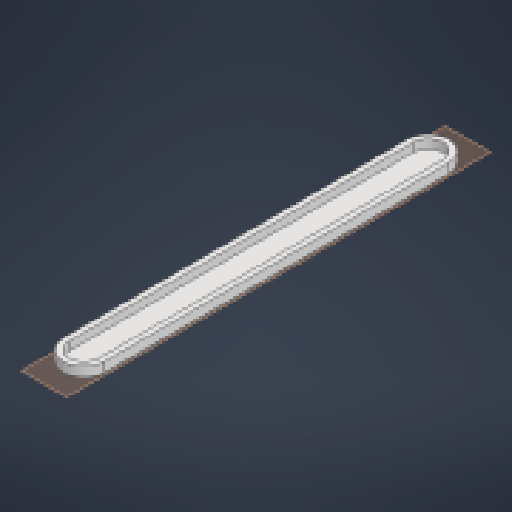
# Autodesk Inventor part: wiper_outside
Saved by Autodesk Inventor 2026.2 (Build 302298000, 298)
## iProperties
Created: 2026-04-07
Part Number: wiper_outside
Material: ABS Plastic
Document SubType Name: Modeling
Designer: Tathagata Sikdar
Density: 1.06 g/cm^3
Appearance: Smooth - White
Author: Tathagata Sikdar
Autodesk Inventor part; units mm, degrees
ref_plane "YZ Plane" through (0, 0, 0) normal (1, 0, 0) x (0, 1, 0)
ref_plane "XZ Plane" through (0, 0, 0) normal (0, 1, 0) x (-1, 0, 0)
ref_plane "XY Plane" through (0, 0, 0) normal (0, 0, 1) x (1, 0, 0)
ref_plane "Work Plane1" through (-54.4323, -35.9721, 73.855) normal (0, 1, 0) x (-1, 0, 0)
sketch "Sketch1" plane through (-54.4323, -35.9721, 73.855) normal (0, 1, 0) x (-1, 0, 0)
  arc A0 (7.2, 60.25) -> (-7.2, 60.25) centre (0, 60.25) ccw projected
  line L0 (-7.2, -60.25) -> (-7.2, 60.25) projected
  arc A1 (-7.2, -60.25) -> (7.2, -60.25) centre (0, -60.25) ccw projected
  line L1 (7.2, 60.25) -> (7.2, -60.25) projected
  arc A2 (-5.2, -60.25) -> (5.2, -60.25) centre (0, -60.25) ccw projected
  line L2 (-5.2, -60.25) -> (-5.2, 60.25) projected
  line L3 (5.2, 60.25) -> (5.2, -60.25) projected
  arc A3 (5.2, 60.25) -> (-5.2, 60.25) centre (0, 60.25) ccw projected
  point P0 (-54.4323, -73.855)
extrude "Extrusion1" add sketch "Sketch1" along normal blind 0.4 contours L1 A1 L0 A0 | L2 A3 L3 A2
sketch "Sketch2" plane through (-54.4323, -35.5721, 73.855) normal (0, 1, 0) x (1, 0, 0)
  arc A0 (-7.2, -60.25) -> (7.2, -60.25) centre (0, -60.25) ccw projected
  line L0 (-7.2, -60.25) -> (-7.2, 60.25) projected
  arc A1 (7.2, 60.25) -> (-7.2, 60.25) centre (0, 60.25) ccw projected
  line L1 (7.2, 60.25) -> (7.2, -60.25) projected
  line L2 (5.2, -60.25) -> (5.2, 60.25) projected
  arc A2 (5.2, 60.25) -> (-5.2, 60.25) centre (0, 60.25) ccw projected
  line L3 (-5.2, 60.25) -> (-5.2, -60.25) projected
  arc A3 (-5.2, -60.25) -> (5.2, -60.25) centre (0, -60.25) ccw projected
  point P0 (54.4323, 73.855)
extrude "Extrusion2" add sketch "Sketch2" along normal blind 3
body "Solid1"
